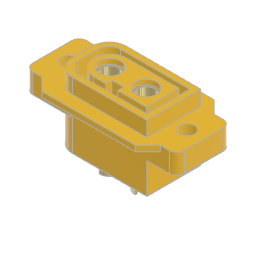
XT60E-F_panel (Autodesk Fusion 360 design; units mm, degrees)
Autodesk Fusion 360 part; units mm, degrees
sketch "Sketch1" plane through (0, 0, 0) normal (0, 0, 1) x (1, 0, 0)
  circle A0 centre (-3.6, 0) radius 1.75
  line L0 (0, 0) -> (-3.6, 0) construction
  line L1 (0, 0) -> (0, 3.25) construction
  circle A1 centre (-3.6, 0) radius 2.15
  circle A2 centre (-3.6, 0) radius 3.25
  circle A3 centre (3.6, 0) radius 2.15
  circle A4 centre (3.6, 0) radius 1.75
  line L2 (-3.6, 3.25) -> (6.95, 3.25)
  line L3 (6.95, 3.25) -> (6.95, -3.25)
  line L4 (6.95, -3.25) -> (-3.6, -3.25)
  line L5 (-6.85, 0) -> (-6.85, 3.25) construction
  line L6 (9.15, 5.375) -> (-5.75, 5.375)
  line L7 (-9.15, 1.975) -> (-9.15, -1.975)
  line L8 (-5.75, -5.375) -> (9.15, -5.375)
  line L9 (9.15, -5.375) -> (9.15, 5.375)
  line L10 (9.15, 5.375) -> (-9.15, -5.375) construction
  line L11 (-9.15, 5.375) -> (9.15, -5.375) construction
  line L12 (-9.15, 1.975) -> (-9.15, 5.375) construction
  line L13 (-5.75, 5.375) -> (-9.15, 5.375) construction
  line L14 (-9.15, -1.975) -> (-9.15, -5.375) construction
  line L15 (-5.75, -5.375) -> (-9.15, -5.375) construction
  arc A5 (-5.75, 5.375) -> (-9.15, 1.975) centre (-5.75, 1.975) ccw
  arc A6 (-9.15, -1.975) -> (-5.75, -5.375) centre (-5.75, -1.975) ccw
  line L16 (-5.75, -1.975) -> (-5.75, 1.975) construction
  line L17 (-5.75, -4.275) -> (8.05, -4.275)
  line L18 (8.05, -4.275) -> (8.05, 4.275)
  line L19 (8.05, 4.275) -> (-5.75, 4.275)
  arc A7 (-5.75, 4.275) -> (-8.05, 1.975) centre (-5.75, 1.975) ccw
  line L20 (-8.05, 1.975) -> (-8.05, -1.975)
  arc A8 (-8.05, -1.975) -> (-5.75, -4.275) centre (-5.75, -1.975) ccw
  line L21 (15.15, 5.375) -> (-15.15, 5.375)
  line L22 (-15.15, 5.375) -> (-15.15, -5.375)
  line L23 (-15.15, -5.375) -> (15.15, -5.375)
  line L24 (15.15, -5.375) -> (15.15, 5.375)
  line L25 (15.15, 5.375) -> (-15.15, -5.375) construction
  line L26 (-15.15, 5.375) -> (15.15, -5.375) construction
  line L27 (0, 0) -> (-11.85, 0) construction
  circle A9 centre (-11.85, 0) radius 1.5
  circle A10 centre (11.85, 0) radius 1.5
  line L28 (-11.85, 0) -> (-11.85, 5.375) construction
  line L29 (-11.85, 5.375) -> (-9.35, 7.875)
  line L30 (-9.35, 7.875) -> (0, 7.875)
  line L31 (9.35, 7.875) -> (0, 7.875)
  line L32 (11.85, 5.375) -> (9.35, 7.875)
  line L33 (-9.35, -7.875) -> (0, -7.875)
  line L34 (-11.85, -5.375) -> (-9.35, -7.875)
  line L35 (9.35, -7.875) -> (0, -7.875)
  line L36 (11.85, -5.375) -> (9.35, -7.875)
  line L37 (1.2, -3.25) -> (-1.2, -3.25)
  line L38 (-1.2, -3.25) -> (-1.2, -2.05)
  line L39 (-1.2, -2.05) -> (1.2, -2.05)
  line L40 (1.2, -2.05) -> (1.2, -3.25)
  line L41 (0, -2.05) -> (0, -3.25) construction
  dimension "d3" = 3.5
  dimension "d5" = 1.85
  dimension "d7" = 4.3
  dimension "d8" = 6.5
  dimension "d9" = 13.8
  dimension "d10" = 1.1
  dimension "d11" = 1.2
  dimension "d12" = 10.75
  dimension "d13" = 18.3
  dimension "d14" = -1.1
  dimension "d15" = 30.3
  dimension "d16" = 3
  dimension "d18" = 1.8
  dimension "d19" = 45
  dimension "d20" = 2.5
  dimension "d33" = 1.2
  dimension "d34" = 2.4
  constraint coincident A0.centre L0.end
  constraint coincident L1.start L0
  constraint coincident L0.start L1.start
  constraint perpendicular L0 L1
  constraint horizontal L0
  constraint concentric A0 A1
  constraint concentric A0 A2
  constraint symmetric A0 L1 A4
  constraint symmetric L1 A1 A3
  constraint coincident A2 L2.start
  constraint tangent A2 L2
  constraint horizontal L2
  constraint perpendicular L2 L3
  constraint coincident A2 L4.end
  constraint tangent A2 L4
  constraint parallel L2 L4
  constraint coincident A2 L5.start
  constraint tangent A2 L5
  constraint perpendicular L2 L5
  constraint coincident L2 L5.end
  constraint horizontal L6
  constraint perpendicular L6 L7
  constraint parallel L6 L8
  constraint parallel L7 L9
  constraint coincident L10 L0.start
  constraint coincident L11 L0.start
  constraint perpendicular L12 L13
  constraint collinear L8 L15
  constraint collinear L7 L12
  constraint coincident L11.start L12.end
  constraint coincident L1.end L2
  constraint tangent L6 A5
  constraint tangent L7 A5
  constraint symmetric L0 L6.end L8.start
  constraint symmetric L0 L7.start L7.end
  constraint symmetric L0 A5 A6
  constraint coincident L8.start L15.start
  constraint coincident L7.end L14.start
  constraint coincident A6.centre L16.start
  constraint coincident A5.centre L16.end
  constraint tangent A1 L16
  constraint horizontal L21
  constraint perpendicular L21 L22
  constraint parallel L21 L23
  constraint parallel L22 L24
  constraint coincident L25 L0.start
  constraint coincident L26 L0.start
  constraint collinear L6 L21
  constraint horizontal L27
  constraint coincident L27.end A9.centre
  constraint symmetric L1 A9 A10
  constraint coincident L21 L28.end
  constraint perpendicular L21 L28
  constraint perpendicular L28 L30
  constraint vertical L0.start L30.end
  constraint symmetric L1 L28.end L32.start
  constraint symmetric L1 L29.end L31.start
  constraint symmetric L1 L30.end L31.end
  constraint symmetric L0 L28.end L34.start
  constraint symmetric L0 L29.end L33.start
  constraint symmetric L0 L30.end L33.end
  constraint symmetric L0 L31.start L35.start
  constraint symmetric L0 L32.start L36.start
  constraint horizontal L37
  constraint vertical L38
  constraint horizontal L39
  constraint vertical L40
  constraint coincident L4 L37.start
  constraint midpoint L39 L41.start
  constraint midpoint L37 L41.end
  constraint collinear L1 L41
  measures "d3" diameter of A0
  measures "d5" distance of A0 L1
  measures "d7" diameter of A1
  measures "d8" diameter of A2
  measures "d9" distance of L3 L5
  measures "d10" distance of A1 L5
  measures "d11" distance of A3 L3
  measures "d12" distance of L6.start L8.end
  measures "d13" distance of L10.end L8.end
  measures "d15" distance of L21.start L21.end
  measures "d16" diameter of A9
  measures "d18" distance of L22 A9
  measures "d19" angle of L21 L29
  measures "d20" distance of L6 L30
  measures "d33" distance of L37.start L39.end
  measures "d34" distance of L38.end L39.end
extrude "Extrude1" add sketch "Sketch1" against normal blind 13.2 contours A2 L38 L39 | A2 L2 L3 L4 L39 L40 | A2 L4 L37 L38 L39 L40 | A2 L38 L39 | A2 L4 L38 | L6 L7 L8 L9 A5 A6 L21 L23 | L17 L18 L19 A7 L20 A8 makes body 1
extrude "Extrude5" cut sketch "Sketch1" against normal blind 9.2 contours A2 L4 L37 L38 L39 L40 | A2 L38 L39 | L17 L18 L19 A7 L20 A8 picked at (-1.1588, -2.0977) bodies 1
extrude "Extrude2" add sketch "Sketch1" against normal blind 4 from surface at -3 contours L9 L21 L23 L24 | L7 A5 A6 L21 L22 L23 bodies 1
extrude "Extrude3" add sketch "Sketch1" against normal blind 1.1 from surface at -3 contours L6 L21 L29 L30 L31 L32 | L8 L23 L33 L34 L35 L36 bodies 1
extrude "Extrude4" add sketch "Sketch1" along normal blind 0.1 contours A2 L38 L39 | A2 L2 L3 L4 L39 L40 | A2 L4 L38 picked at (-1.6616, -2.0776) bodies 1
extrude "Extrude6" cut sketch "Sketch1" along normal blind 2 from surface at -13.2 contours A2 L38 L39 | A2 L2 L3 L4 L39 L40 | A2 L4 L37 L38 L39 L40 | A2 L38 L39 | A2 L4 L38 bodies 1
sketch "Sketch2" plane through (0, 0, -11.2) normal (0, 0, -1) x (1, 0, 0)
  line L0 (6.95, 3.25) -> (-3.6, 3.25)
  arc A0 (-3.6, 3.25) -> (-3.6, -3.25) centre (-3.6, 0) ccw
  line L1 (-3.6, -3.25) -> (6.95, -3.25)
  line L2 (6.95, -3.25) -> (6.95, 3.25)
  circle A1 centre (3.6, 0) radius 2.15
  circle A2 centre (-3.6, 0) radius 2.15
  line L3 (0.375, 3.25) -> (-0.375, 3.25)
  line L4 (-0.375, 3.25) -> (-0.375, -3.25)
  line L5 (-0.375, -3.25) -> (0.375, -3.25)
  line L6 (0.375, -3.25) -> (0.375, 3.25)
  line L7 (0.375, 3.25) -> (-0.375, -3.25) construction
  line L8 (-0.375, 3.25) -> (0.375, -3.25) construction
  dimension "d38" = 0.75
  constraint horizontal L3
  constraint perpendicular L3 L4
  constraint parallel L3 L5
  constraint parallel L4 L6
  constraint coincident L0 L3.start
  constraint coincident L7 origin
  constraint coincident L8 origin
  measures "d38" distance of L4.end L5.end
extrude "Extrude7" add sketch "Sketch2" along normal blind 2 contours L0 L1 L3 L4 L5 L6 bodies 1
fillet "Fillet1" radius 1.5 4 edges at (15.15, -5.375, -5) (15.15, 5.375, -5) (-15.15, 5.375, -5) (-15.15, -5.375, -5) on bodies 1
sketch "Sketch1 (2)" plane through (0, 0, 0.1) normal (0, 0, 1) x (-1, 0, 0) in component "pins"
  circle A0 centre (3.6, 0) radius 2.15
  circle A1 centre (-3.6, 0) radius 2.15
  line L0 (1.2, 3.25) -> (1.2, 2.05)
  line L1 (1.2, 2.05) -> (-1.2, 2.05)
  line L2 (-1.2, 2.05) -> (-1.2, 3.25)
  line L3 (-1.2, 3.25) -> (-6.95, 3.25)
  line L4 (-6.95, 3.25) -> (-6.95, -3.25)
  line L5 (-6.95, -3.25) -> (3.6, -3.25)
  arc A2 (3.6, -3.25) -> (3.6, 3.25) centre (3.6, 0) ccw
  line L6 (3.6, 3.25) -> (1.2, 3.25)
  circle A3 centre (3.6, 0) radius 1.75
  circle A4 centre (-3.6, 0) radius 1.75
  dimension "d41" = 3.5
  dimension "d42" = 3.5
  constraint concentric A0 A3
  constraint concentric A1 A4
  measures "d41" diameter of A3
  measures "d42" diameter of A4
extrude "Extrude1'" add sketch "Sketch1 (2)" against normal blind 16.4 from surface at -1 separate body contours A0 | A1 makes body 2 at (1.4607, 0.2141, -6.3667) makes body 3 at (-5.7393, 0.2141, -6.3667) in component "pins"
sketch "Sketch2 (2)" plane through (0, 0, -17.3) normal (0, 0, -1) x (1, 0, 0) in component "pins"
  circle A0 centre (-3.6, 0) radius 1.75
  circle A1 centre (-3.6, 0) radius 2.15
  line L0 (-3.6, 2.15) -> (-3.6, -2.15)
  circle A2 centre (3.6, 0) radius 2.15
  line L1 (3.6, 2.15) -> (3.6, -2.15)
  circle A3 centre (3.6, 0) radius 1.75
  constraint coincident A1 L0.start
  constraint vertical L0
  constraint coincident A0.centre L0
  constraint coincident A1 L0.end
  constraint coincident A2 L1.start
  constraint vertical L1
  constraint coincident A2 L1.end
  constraint coincident A2.centre L1
extrude "Extrude2'" cut sketch "Sketch2 (2)" against normal blind 2.9 contours A0 A1 L0 | A2 L1 A3 picked at (-3.7938, 2.0021) picked at (3.702, 2.0094) bodies 2 3 in component "pins"
extrude "Extrude3'" add sketch "Sketch1 (2)" against normal blind 3 from surface at -10 contours A3 | A4 bodies 2 3 in component "pins"
fillet "Fillet1'" radius 1.75 4 edges at (5.2316, 0.6328, -12.9) (5.2316, -0.6328, -9.9) (-1.9684, 0.6328, -12.9) (-1.9684, -0.6328, -9.9) on bodies 2 3 in component "pins"
sketch "Sketch1 (3)" plane through (0, 0, -7) normal (0, 0, -1) x (1, 0, 0) in component "nuts"
  arc A0 (13.65, -5.375) -> (15.15, -3.875) centre (13.65, -3.875) ccw
  line L0 (15.15, -3.875) -> (15.15, 3.875)
  arc A1 (15.15, 3.875) -> (13.65, 5.375) centre (13.65, 3.875) ccw
  line L1 (13.65, 5.375) -> (9.15, 5.375)
  line L2 (9.15, 5.375) -> (9.15, -5.375)
  line L3 (9.15, -5.375) -> (13.65, -5.375)
  circle A2 centre (11.85, 0) radius 1.5
  line L4 (14.3, 1.4145) -> (11.85, 2.829)
  line L5 (11.85, 2.829) -> (9.4, 1.4145)
  line L6 (9.4, 1.4145) -> (9.4, -1.4145)
  line L7 (9.4, -1.4145) -> (11.85, -2.829)
  line L8 (11.85, -2.829) -> (14.3, -1.4145)
  line L9 (14.3, -1.4145) -> (14.3, 1.4145)
  line L10 (0, 0) -> (0, 2.829) construction
  line L11 (-9.4, 1.4145) -> (-9.4, -1.4145)
  line L12 (-9.4, -1.4145) -> (-11.85, -2.829)
  line L13 (-11.85, -2.829) -> (-14.3, -1.4145)
  line L14 (-14.3, -1.4145) -> (-14.3, 1.4145)
  line L15 (-14.3, 1.4145) -> (-11.85, 2.829)
  line L16 (-11.85, 2.829) -> (-9.4, 1.4145)
  circle A3 centre (11.85, 0) radius 1.25
  circle A4 centre (-11.85, 0) radius 1.25
  point P0 (11.85, 0)
  dimension "d55" = 2.45
  dimension "d56" = 2.5
  constraint coincident P0 A2.centre
  constraint parallel L0 L9
  constraint coincident L10.start origin
  constraint vertical L10
  constraint horizontal L4.end L10.end
  constraint symmetric L4.start L10 L14.end
  constraint symmetric L4.end L10 L15.end
  constraint symmetric L5.end L10 L11.start
  constraint symmetric L6.end L10 L11.end
  constraint symmetric L7.end L10 L12.end
  constraint symmetric L8.end L10 L13.end
  constraint symmetric L10 A3 A4
  measures "d55" distance of P0 L9
  measures "d56" diameter of A3
extrude "Extrude8" cut sketch "Sketch1 (3)" against normal blind 2 contours A2 | L4 L5 L6 L7 L8 L9 | L11 L12 L13 L14 L15 L16 bodies 1
extrude "Extrude1''" add sketch "Sketch1 (3)" against normal blind 2 separate body contours A2 | L4 L5 L6 L7 L8 L9 | L11 L12 L13 L14 L15 L16 makes body 4 at (12.875, 1.7754, -7) makes body 5 at (-12.875, 1.7754, -7) in component "nuts"
chamfer "Chamfer1" distance 0.2 angle 45 4 faces at (-12.875, 1.7754, -7) (-12.875, 1.7754, -5) (12.875, 1.7754, -7) (12.875, 1.7754, -5) on bodies 4 5 in component "nuts"
component "pins" placed x (1, 0, 0) y (0, 1, 0) z (0, 0, 1) at (0, 0, 0)
component "nuts" placed x (1, 0, 0) y (0, 1, 0) z (0, 0, 1) at (0, 0, 0)
equation "d5 = ( 3.7 / 2 ) * 1 mm"
equation "d55 = ( 4.9 / 2 ) * 1 mm"
named bodies: "housing"
